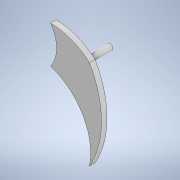
# Autodesk Inventor part: iris bottom chip
Saved by Autodesk Inventor 2021 (Build 250183000, 183)
## iProperties
Created: 2020-07-09
Part Number: iris bottom chip
Material: Generic
Document SubType Name: Modeling
Designer: saipr
Density: 1 g/cm^3
Appearance: Default
Author: saipr
Autodesk Inventor part; units mm, degrees
ref_plane "YZ Plane" through (0, 0, 0) normal (1, 0, 0) x (0, 1, 0)
ref_plane "XZ Plane" through (0, 0, 0) normal (0, 1, 0) x (-1, 0, 0)
ref_plane "XY Plane" through (0, 0, 0) normal (0, 0, 1) x (1, 0, 0)
sketch "Sketch2" plane through (0, 0, 0) normal (0, 0, 1) x (1, 0, 0)
  arc A0 (40.01, -31.3024) -> (31.3024, 40.01) centre (0, 0) ccw
  circle A1 centre (0, 0) radius 50.8
  circle A2 centre (0, 0) radius 25.4
  line L0 (0, 0) -> (43.9941, 25.4)
  line L1 (0, 0) -> (50.8, 0)
  line L2 (0, 0) -> (43.9941, -25.4)
  arc A3 (43.9941, -25.4) -> (21.997, 12.7) centre (11.6686, -18.6631) ccw
  line L3 (0, 0) -> (0, 50.8)
  arc A4 (43.9941, 25.4) -> (0, 25.4) centre (21.997, 0.7738) ccw
  arc A5 (43.9941, 25.4) -> (21.997, 33.7938) centre (21.997, 0.7738) ccw
  arc A6 (21.997, 12.7) -> (21.997, 33.7938) centre (7.4101, 23.2469) ccw
  line L4 (43.9941, 25.4) -> (41.2445, 23.8125)
  line L5 (41.2445, 23.8125) -> (38.4948, 22.225)
  circle A7 centre (39.8696, 23.0188) radius 1.5875
  line L6 (0, 0) -> (-43.9941, 25.4)
  arc A8 (0, 50.8) -> (-21.997, 12.7) centre (10.3284, 19.4369) ccw
  dimension "d97" = 50.8
  dimension "d102" = 50.8
  dimension "d121" = 30
  dimension "d122" = 60
  dimension "d123" = 33.02
  dimension "d127" = 33.02
  dimension "d130" = 3.175
  dimension "d131" = 3.175
  dimension "d134" = 60
  dimension "d135" = 33.02
  constraints: 18 point on circle, 14 end point, 8 centre point, 4 midpoint, 3 coincident, 3 point on line, 2 concentric, 1 horizontal, 1 vertical, 3 other
  measures "d97" radius of A0
  measures "d102" diameter of A2
  measures "d121" angle of L1 L0
  measures "d122" angle of L0 L2
  measures "d123" radius of A3
  measures "d127" radius of A4
  measures "d130" distance of L4.start L4.end
  measures "d131" distance of L4.end L5.end
  measures "d134" angle of L3 L6
  measures "d135" radius of A8
extrude "Extrusion8" add sketch "Sketch2" along normal blind 3.175 contours A3 L1 A0 | L1 A3 L0 A7 A0 | L0 A7 A6 A4 | A7 L0 | L0 A7
extrude "Extrusion9" add sketch "Sketch2" against normal blind 12.7 contours A7 L0 | L0 A7
equation "\"d135\" = d123"
body "Solid4"
